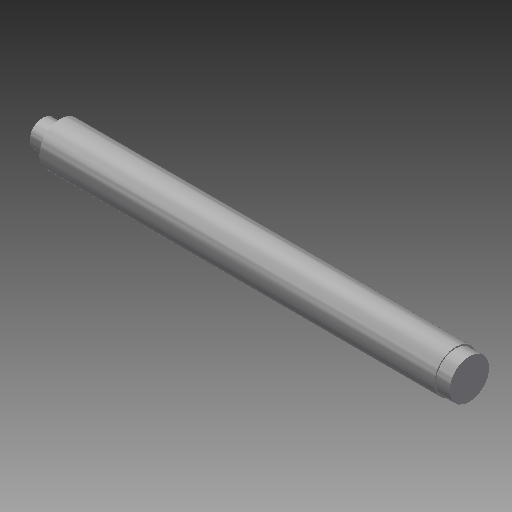
# Autodesk Inventor part: Shaft
Saved by Autodesk Inventor 2019.4 (Build 234330000, 330)
## iProperties
Created: 2020-01-03
Part Number: Shaft
Material: Steel
Document SubType Name: Modeling
Designer: Mark
Density: 7.85 g/cm^3
Appearance: Steel
Mass: 250.238 g
Surface Area: 84.7162 cm^2
Volume: 31.8774 cm^3
CustomPartVersion: 1
Length: 161.500 mm
Author: Mark
Autodesk Inventor part; units mm, degrees
ref_plane "Start Plane" through (0, 0, 0) normal (1, 0, 0) x (0, 1, 0)
ref_plane "XZ Plane" through (0, 0, 0) normal (0, 1, 0) x (-1, 0, 0)
ref_plane "XY Plane" through (0, 0, 0) normal (0, 0, 1) x (1, 0, 0)
sketch "Main Sketch" plane through (0, 0, 0) normal (0, 0, 1) x (1, 0, 0)
  line L0 (0, 0) -> (161.5, 0)
  line L1 (0, 0) -> (0, 5)
  line L2 (6.7, 5) -> (6.7, 8)
  line L3 (0, 5) -> (6.7, 5)
  line L4 (156.3, 8) -> (156.3, 7.5)
  line L5 (6.7, 8) -> (156.3, 8)
  line L6 (161.5, 7.5) -> (161.5, 0)
  line L7 (156.3, 7.5) -> (161.5, 7.5)
  dimension "d3" = 10
  dimension "d5" = 16
  dimension "d6" = 15
  constraints: 16 end point, 4 vertical, 2 horizontal
  measures "d3" diameter of L3 L0
  measures "d5" diameter of L5 L0
  measures "d6" diameter of L7 L0
revolve "Revolution1" add sketch "Main Sketch" angle 360 about axis through (0, 0, 0) along (1, 0, 0)
equation "\"Length\" = 161.5"
body "Solid1"
